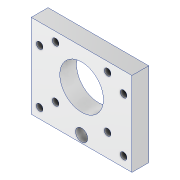
# Autodesk Inventor part: Techo Espaciador
Saved by Autodesk Inventor 2020 (Build 240168000, 168)
## iProperties
Created: 2020-05-16
Part Number: Techo Espaciador
Material: Aluminum 6061
Document SubType Name: Modeling
Designer: Dante
Density: 2.7 g/cm^3
Appearance: Aluminum - Flat
Mass: 63.9506 g
Surface Area: 87.592 cm^2
Volume: 23.6854 cm^3
Author: Dante
Autodesk Inventor part; units mm, degrees
ref_plane "YZ Plane" through (0, 0, 0) normal (1, 0, 0) x (0, 1, 0)
ref_plane "XZ Plane" through (0, 0, 0) normal (0, 1, 0) x (-1, 0, 0)
ref_plane "XY Plane" through (0, 0, 0) normal (0, 0, 1) x (1, 0, 0)
sketch "Sketch1" plane through (0, 0, 0) normal (0, 0, 1) x (1, 0, 0)
  line L0 (0, 0) -> (0, -50)
  line L1 (0, -50) -> (60, -50)
  line L2 (60, -50) -> (60, 0)
  line L3 (60, 0) -> (0, 0)
  circle A0 centre (5, -12) radius 2
  circle A1 centre (5, -44) radius 2
  circle A2 centre (55, -12) radius 2
  circle A3 centre (55, -44) radius 2
  line L4 (9, 0) -> (9, -42)
  line L5 (9, -42) -> (51, -42)
  line L6 (51, -42) -> (51, 0)
  line L7 (51, 0) -> (9, 0)
  circle A4 centre (30, -21) radius 13
  circle A5 centre (14.5, -5.5) radius 2
  circle A6 centre (14.5, -36.5) radius 2
  circle A7 centre (45.5, -36.5) radius 2
  circle A8 centre (45.5, -5.5) radius 2
  circle A9 centre (30, -45.75) radius 3.625
  dimension "d0" = 50
  dimension "d1" = 60
  dimension "d2" = 4
  dimension "d3" = 4
  dimension "d4" = 4
  dimension "d5" = 4
  dimension "d6" = 5
  dimension "d7" = 5
  dimension "d8" = 5
  dimension "d9" = 5
  dimension "d11" = 6
  dimension "d13" = 6
  dimension "d16" = 42
  dimension "d17" = 42
  dimension "d18" = 42
  dimension "d19" = 26
  dimension "d20" = 21
  dimension "d21" = 30
  dimension "d22" = 21
  dimension "d23" = 21
  dimension "d24" = 4
  dimension "d25" = 4
  dimension "d26" = 4
  dimension "d27" = 4
  dimension "d28" = 31
  dimension "d29" = 31
  dimension "d30" = 31
  dimension "d31" = 31
  dimension "d32" = 5.5
  dimension "d33" = 5.5
  dimension "d34" = 5.5
  dimension "d35" = 5.5
  dimension "d40" = 38
  dimension "d41" = 38
  dimension "d42" = 7.25
  dimension "d43" = 4.25
  constraints: 16 end point, 10 centre point, 4 perpendicular, 2 vertical, 1 horizontal
  measures "d0" distance of L0.start L0.end
  measures "d1" distance of L0.end L1.end
  measures "d2" diameter of A0
  measures "d3" diameter of A1
  measures "d4" diameter of A2
  measures "d5" diameter of A3
  measures "d6" distance from line of L0 A0.centre
  measures "d7" distance from line of L0 A1.centre
  measures "d8" distance from line of L2 A2.centre
  measures "d9" distance from line of A3.centre L2
  measures "d11" distance from line of L1 A3.centre
  measures "d13" distance from line of L1 A1.centre
  measures "d16" distance of L4.start L4.end
  measures "d17" distance of L4.end L5.end
  measures "d18" distance of L5.end L6.end
  measures "d19" diameter of A4
  measures "d20" distance from line of L6 A4.centre
  measures "d21" distance from line of A4.centre L2
  measures "d22" distance from line of L3 A4.centre
  measures "d23" distance from line of L7 A4.centre
  measures "d24" diameter of A5
  measures "d25" diameter of A6
  measures "d26" diameter of A7
  measures "d27" diameter of A8
  measures "d28" distance of A5.centre A8.centre
  measures "d29" distance of A8.centre A7.centre
  measures "d30" distance of A5.centre A6.centre
  measures "d31" distance of A6.centre A7.centre
  measures "d32" distance from line of L4 A5.centre
  measures "d33" distance from line of L4 A6.centre
  measures "d34" distance from line of L5 A6.centre
  measures "d35" distance from line of L3 A8.centre
  measures "d40" distance from line of A2.centre L1
  measures "d41" distance from line of A0.centre L1
  measures "d42" diameter of A9
  measures "d43" distance from line of L1 A9.centre
extrude "Extrusion3" add sketch "Sketch1" along normal blind 10
body "Solid2"
